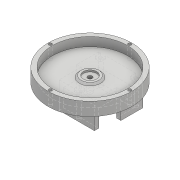
# Autodesk Inventor part: arm_0_bottom
Saved by Autodesk Inventor 2018 (Build 220112000, 112)
## iProperties
Created: 2017-12-03
Part Number: arm_0_bottom
Material: Generic
Document SubType Name: Modeling
Designer: Bardo91
Density: 1 g/cm^3
Appearance: Default
Author: Bardo91
Autodesk Inventor part; units mm, degrees
ref_plane "YZ Plane" through (0, 0, 0) normal (1, 0, 0) x (0, 1, 0)
ref_plane "XZ Plane" through (0, 0, 0) normal (0, 1, 0) x (-1, 0, 0)
ref_plane "XY Plane" through (0, 0, 0) normal (0, 0, 1) x (1, 0, 0)
sketch "Sketch1" plane through (0, 0, 0) normal (0, 0, 1) x (1, 0, 0)
  circle A0 centre (0, 0) radius 47.5
  dimension "d0" = 95
  constraints: 1 centre point, 1 coincident
  measures "d0" diameter of A0
extrude "base" add sketch "Sketch1" along normal blind 5
sketch "Sketch2" plane through (0, 0, 5) normal (0, 0, 1) x (1, 0, 0)
  circle A0 centre (0, 0) radius 47.5
  circle A1 centre (0, 0) radius 42.5
  dimension "d3" = 95
  dimension "d4" = 85
  constraints: 2 centre point, 2 coincident
  measures "d3" diameter of A0
  measures "d4" diameter of A1
extrude "wall" add sketch "Sketch2" along normal blind 10
sketch "Sketch3" plane through (0, 0, 5) normal (0, 0, 1) x (1, 0, 0)
  circle A0 centre (0, 0) radius 7.5
  circle A1 centre (0, 0) radius 10
  dimension "d7" = 15
  dimension "d8" = 20
  constraints: 2 centre point, 2 coincident
  measures "d7" diameter of A0
  measures "d8" diameter of A1
extrude "servo_horn_place" add sketch "Sketch3" along normal blind 2
chamfer "Chamfer1" distance 2 angle 45 1 edges at (-10, 0, 5)
sketch "Sketch4" plane through (0, 0, 5) normal (0, 0, 1) x (1, 0, 0)
  circle A0 centre (0, 0) radius 2.5
  dimension "d15" = 5
  constraints: 1 centre point, 1 coincident
  measures "d15" diameter of A0
extrude "servo_horn_screw_hole" cut sketch "Sketch4" against normal through all
sketch "Sketch5" plane through (0, 0, 15) normal (0, 0, 1) x (1, 0, 0)
  line L0 (0, 0) -> (45, 0)
  circle A0 centre (45, 0) radius 1.75
  circle A1 centre (0, 45) radius 1.75
  circle A2 centre (-45, 0) radius 1.75
  circle A3 centre (0, -45) radius 1.75
  dimension "d18" = 45
  dimension "d19" = 3.5
  dimension "d22" = 360
  constraints: 4 centre point, 2 end point, 1 coincident, 1 horizontal, 9 other
  measures "d18" distance of L0.start L0.end
  measures "d19" diameter of A0
extrude "attach_case" cut sketch "Sketch5" against normal through all
sketch "Sketch6" plane through (0, 0, 0) normal (0, 0, -1) x (-1, 0, 0)
  line L0 (0, 0) -> (20, 0)
  line L1 (20, 0) -> (20, -10)
  line L2 (20, -10) -> (-20, -10)
  line L3 (-20, -10) -> (-20, 10)
  line L4 (-20, 30) -> (20, 30)
  line L5 (20, 30) -> (20, 0)
  line L6 (-20, -10) -> (-20, -15)
  line L7 (-20, -15) -> (-25, -15)
  line L8 (-25, -15) -> (-25, -10)
  line L9 (-25, 35) -> (25, 35)
  line L10 (25, 35) -> (25, 10)
  line L11 (25, -15) -> (20, -15)
  line L12 (20, -10) -> (20, -15)
  line L13 (20, -10) -> (20, 0)
  line L14 (20, 10) -> (25, 10)
  line L15 (-20, 10) -> (-25, 10)
  line L16 (20, -15) -> (-20, -15)
  line L17 (20, 0) -> (20, 10)
  line L18 (25, 10) -> (25, -15)
  line L19 (-20, 10) -> (-20, 30)
  line L20 (-25, 10) -> (-25, 35)
  line L21 (-25, -10) -> (-25, 10)
  dimension "d26" = 20
  dimension "d27" = 10
  dimension "d28" = 40
  dimension "d29" = 40
  dimension "d30" = 40
  dimension "d31" = 5
  dimension "d32" = 5
  dimension "d33" = 50
  dimension "d34" = 50
  dimension "d39" = 20
  constraints: 44 end point, 14 perpendicular, 4 point on line, 2 collinear, 2 vertical, 1 horizontal
  measures "d26" distance of L0.start L0.end
  measures "d27" distance of L0.end L1.end
  measures "d28" distance of L1.end L2.end
  measures "d29" distance of L2.end L4.start
  measures "d30" distance of L4.start L4.end
  measures "d31" distance of L2.end L6.end
  measures "d32" distance of L6.end L7.end
  measures "d33" distance of L7.end L9.start
  measures "d34" distance of L9.start L9.end
  measures "d39" distance of L1.end L14.start
extrude "servo_place" add sketch "Sketch6" along normal blind 30 contours L12 L16 L6 L2 | L5 L4 L19 L15 L20 L9 L10 L14
sketch "Sketch7" plane through (0, 0, 0) normal (0, 0, -1) x (-1, 0, 0)
  line L0 (20, -10) -> (-20, -10) projected
  line L1 (-20, 10) -> (-20, -15) projected
  line L2 (20, -10) -> (-20, -10)
  line L3 (-20, -10) -> (-20, 30)
  line L4 (-20, 30) -> (20, 30)
  line L5 (20, 30) -> (20, -10)
  circle A0 centre (0, 0) radius 2.5
  constraints: 8 end point, 2 parallel, 1 centre point, 1 coincident, 1 horizontal, 1 perpendicular
extrude "servo_bed" add sketch "Sketch7" along normal blind 10
sketch "Sketch8" plane through (0, 0, -30) normal (0, 0, -1) x (-1, 0, 0)
  line L0 (-20, -15) -> (20, -15) projected
  line L1 (0, -15) -> (0, -12.5)
  circle A0 centre (0, -12.5) radius 1.75
  line L2 (-25, 35) -> (25, 35) projected
  line L3 (-25, 35) -> (-20, 35)
  line L4 (-20, 35) -> (-20, 32.5)
  line L5 (25, 35) -> (20, 35)
  line L6 (20, 35) -> (20, 32.5)
  circle A1 centre (20, 32.5) radius 1.75
  circle A2 centre (-20, 32.5) radius 1.75
  point P0 (0, 0)
  dimension "d40" = 2.5
  dimension "d41" = 3.5
  dimension "d42" = 5
  dimension "d43" = 2.5
  dimension "d44" = 5
  dimension "d45" = 2.5
  dimension "d46" = 3.5
  dimension "d47" = 3.5
  constraints: 10 end point, 3 centre point, 3 coincident, 2 perpendicular, 2 point on line, 1 midpoint, 1 vertical
  measures "d40" distance of L1.start L1.end
  measures "d41" diameter of A0
  measures "d42" distance of L2.start L3.end
  measures "d43" distance of L3.end L4.end
  measures "d44" distance of L2.end L5.end
  measures "d45" distance of L5.end L6.end
  measures "d46" diameter of A1
  measures "d47" diameter of A2
extrude "screw_holes" cut sketch "Sketch8" against normal up to surface (30 mm away)
sketch "Sketch9" plane through (-25, 35, 0) normal (0, 1, 0) x (1, 0, 0)
  line L0 (0, 0) -> (0, 30) projected
  line L1 (0, 0) -> (5, 0)
  line L2 (72.5, 0) -> (-22.5, 0) projected
  line L3 (5, 0) -> (5, 3)
  line L4 (5, 3) -> (2, 3)
  line L5 (2, 3) -> (2, 0)
  line L6 (2, 0) -> (8, 0)
  line L7 (8, 0) -> (8, 3)
  line L8 (8, 3) -> (5, 3)
  line L9 (50, 0) -> (50, 30) projected
  line L10 (45, 0) -> (50, 0) projected
  line L11 (50, 0) -> (45, 0)
  line L12 (45, 0) -> (45, 3)
  line L13 (45, 0) -> (45, 10) projected
  line L14 (45, 3) -> (48, 3)
  line L15 (48, 3) -> (48, 0)
  line L16 (48, 0) -> (42, 0)
  line L17 (42, 0) -> (42, 3)
  line L18 (42, 3) -> (45, 3)
  point P0 (25, 0)
  dimension "d50" = 5
  dimension "d51" = 3
  dimension "d52" = 3
  dimension "d53" = 6
  dimension "d54" = 5
  dimension "d55" = 3
  dimension "d56" = 3
  dimension "d57" = 6
  constraints: 28 end point, 7 perpendicular, 4 point on line, 2 vertical, 1 horizontal, 5 other
  measures "d50" distance of L0.start L1.end
  measures "d51" distance of L1.end L3.end
  measures "d52" distance of L3.end L4.end
  measures "d53" distance of L5.end L6.end
  measures "d54" distance of L9.start L10.start
  measures "d55" distance of L10.start L12.end
  measures "d56" distance of L12.end L14.end
  measures "d57" distance of L15.end L16.end
extrude "nut_holes_1" cut sketch "Sketch9" against normal blind 6
sketch "Sketch10" plane through (-20, -15, 0) normal (0, -1, 0) x (1, 0, 0)
  line L0 (20, 0) -> (17, 0)
  line L1 (-27.5, 0) -> (67.5, 0) projected
  line L2 (17, 0) -> (17, -3)
  line L3 (17, -3) -> (23, -3)
  line L4 (23, -3) -> (23, 0)
  line L5 (23, 0) -> (20, 0)
  dimension "d60" = 3
  dimension "d61" = 3
  dimension "d62" = 6
  constraints: 10 end point, 4 perpendicular, 2 point on line
  measures "d60" distance of L0.start L0.end
  measures "d61" distance of L0.end L2.end
  measures "d62" distance of L2.end L3.end
extrude "nut_holes_2" cut sketch "Sketch10" against normal blind 6
equation "\"d52\" = 0.5 * d53"
equation "\"d55\" = d51"
equation "\"d56\" = d52"
equation "\"d57\" = d53"
body "Solid1"
